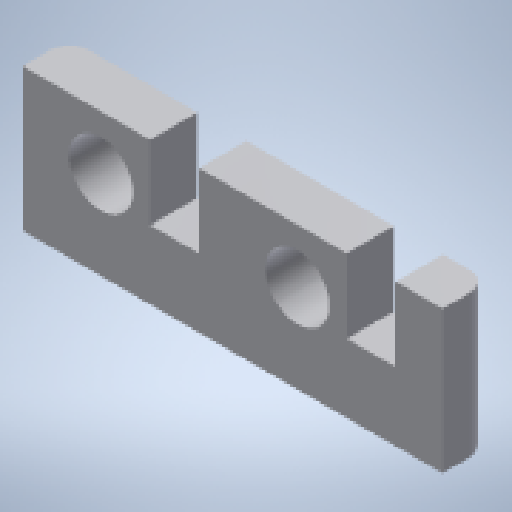
# Autodesk Inventor part: SMASpacer
Saved by Autodesk Inventor 2023.1 (Build 271208000, 208)
## iProperties
Created: 2022-06-15
Part Number: SMASpacer
Material: Generisch
Document SubType Name: Modeling
Designer: pd
Density: 1 g/cm^3
Appearance: Vorgabe
Author: pd
Autodesk Inventor part; units mm, degrees
ref_plane "YZ Plane" through (0, 0, 0) normal (1, 0, 0) x (0, 1, 0)
ref_plane "XZ Plane" through (0, 0, 0) normal (0, 1, 0) x (-1, 0, 0)
ref_plane "Arbeitsebene1" through (-16, -2, -4.8) normal (0, 0, 1) x (1, 0, 0)
sketch "Skizze1" plane through (0, 0, 0) normal (0, 0, 1) x (1, 0, 0)
  line L0 (21.375, -7.25) -> (-21.375, -7.25)
  line L1 (-21.375, -7.25) -> (-21.375, 7.25)
  line L2 (-21.375, 7.25) -> (21.375, 7.25)
  line L3 (21.375, 7.25) -> (21.375, -7.25)
  line L4 (21.375, -7.25) -> (-21.375, 7.25) construction
  line L5 (-21.375, -7.25) -> (21.375, 7.25) construction
  point P0 (0, 0)
  dimension "d0" = 42.75
  dimension "d1" = 14.5
  constraints: 12 end point, 2 midpoint, 2 parallel, 1 horizontal, 1 perpendicular
  measures "d0" distance of L1.end L2.end
  measures "d1" distance of L0.end L1.end
extrude "Extrusion1" add sketch "Skizze1" against normal up to surface (4.8 mm away)
sketch "Skizze2" plane through (0, 0, 0) normal (0, 0, 1) x (1, 0, 0)
  circle A0 centre (-13.375, 1.75) radius 3.25 construction
  circle A1 centre (6.625, 1.75) radius 3.25 construction
  line L0 (-8.124, 7.249) -> (-8.124, -0.049) construction
  line L1 (-3.626, -0.049) -> (-3.626, 7.249) construction
  line L2 (-8.125, -0.05) -> (-3.625, -0.05) construction
  line L3 (11.875, -0.05) -> (16.375, -0.05) construction
  line L4 (16.374, -0.049) -> (16.374, 7.249) construction
  line L5 (11.876, 7.249) -> (11.876, -0.049) construction
  circle A2 centre (6.625, 1.75) radius 3.25
  circle A3 centre (-13.375, 1.75) radius 3.25
  line L6 (16.374, -0.049) -> (11.876, 7.249) construction
  line L7 (11.876, -0.049) -> (16.374, 7.249) construction
  line L8 (-3.625, -0.05) -> (-8.124, 7.2496) construction
  line L9 (-8.125, -0.05) -> (-3.626, 7.249) construction
  line L10 (16.625, 7.6562) -> (11.625, -0.4562) construction
  line L11 (11.625, 7.6562) -> (16.625, -0.4562) construction
  line L12 (-8.3755, 7.4745) -> (-3.3755, 7.4745)
  line L13 (-3.3755, 7.4745) -> (-3.3755, -0.2755)
  line L14 (-3.3755, -0.2755) -> (-8.3755, -0.2755)
  line L15 (-8.3755, -0.2755) -> (-8.3755, 7.4745)
  line L16 (-8.3755, 7.4745) -> (-3.3755, -0.2755) construction
  line L17 (-3.3755, 7.4745) -> (-8.3755, -0.2755) construction
  line L18 (16.625, 7.475) -> (11.625, 7.475)
  line L19 (11.625, 7.475) -> (11.625, -0.275)
  line L20 (11.625, -0.275) -> (16.625, -0.275)
  line L21 (16.625, -0.275) -> (16.625, 7.475)
  line L22 (16.625, 7.475) -> (11.625, -0.275) construction
  line L23 (11.625, 7.475) -> (16.625, -0.275) construction
  point P0 (0, 0)
  point P1 (14.125, 3.6)
  point P2 (-5.8755, 3.5995)
  dimension "d4" = 6.5
  dimension "d5" = 6.5
  dimension "d7" = 5
  dimension "d9" = 7.75
  dimension "d10" = 5
  dimension "d11" = 7.75
  constraints: 36 end point, 8 midpoint, 5 parallel, 2 centre point, 2 coincident, 2 horizontal, 2 perpendicular, 2 point on line
  measures "d4" diameter of A2
  measures "d5" diameter of A3
  measures "d7" distance of L13.end L14.end
  measures "d9" distance of L12.end L13.end
  measures "d10" distance of L20.end L19.end
  measures "d11" distance of L19.end L18.end
extrude "Extrusion2" cut sketch "Skizze2" against normal through all
fillet "Rundung1" radius 2 3 edges at (21.375, 0, -4.8) (0, -7.25, -4.8) (-21.375, 0, -4.8)
